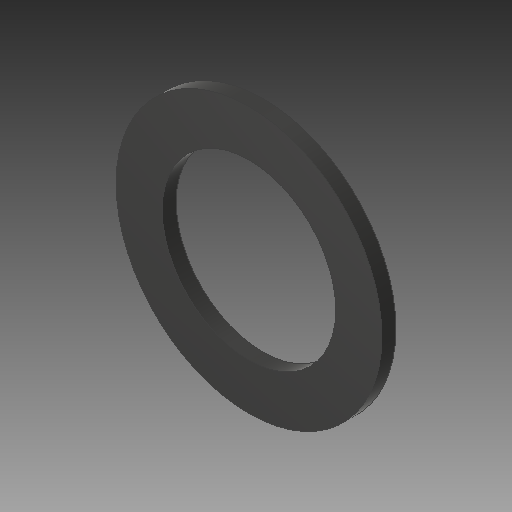
# Autodesk Inventor part: ポリスライダ 内径6 厚み0.5
Saved by Autodesk Inventor 2017.3 (Build 213256000, 256)
## iProperties
Part Number: ポリスライダ 内径6 厚み0.5
Material: アセタール樹脂、黒
Document SubType Name: Modeling
Designer: user
Density: 1.425 g/cm^3
Appearance: 滑らか - 黒
Mass: 0.0289927 g
Surface Area: 1.06044 cm^2
Volume: 0.0203457 cm^3
Author: user
Autodesk Inventor part; units mm, degrees
ref_plane "YZ Plane" through (0, 0, 0) normal (1, 0, 0) x (0, 1, 0)
ref_plane "XZ Plane" through (0, 0, 0) normal (0, 1, 0) x (-1, 0, 0)
ref_plane "XY Plane" through (0, 0, 0) normal (0, 0, 1) x (1, 0, 0)
sketch "スケッチ1" plane through (0, 0, 0) normal (0, 0, 1) x (1, 0, 0)
  circle A0 centre (0, 0) radius 3.1
  circle A1 centre (0, 0) radius 4.75
  dimension "d0" = 6.2
  dimension "d1" = 9.5
  constraints: 2 centre point, 2 coincident
  measures "d0" diameter of A0
  measures "d1" diameter of A1
extrude "押し出し1" add sketch "スケッチ1" along normal blind 0.5
